Autodesk Fusion 360 part; units mm, degrees
note: some values were not read from the file. Set by a fixed rule: which sketch regions a step uses.
(part 4 of 7)
sketch "Sketch76" plane through (0, 116.2145, -31.1396) normal (0, 0.965926, -0.258819) x (-1, 0, 0)
  line L0 (-35.9419, 179.9959) -> (-35.9419, 150.9959)
  line L1 (-35.9419, 150.9959) -> (-72.9419, 150.9959)
  line L2 (-72.9419, 150.9959) -> (-72.9419, 179.9959)
  line L3 (-72.9419, 179.9959) -> (-35.9419, 179.9959)
  line L4 (-30, -37.2933) -> (-30, -46.5838)
  line L5 (-30, -46.5838) -> (22.741, -46.5838)
  ellipse E0 centre (22.741, -39.3535) end of major axis (22.741, -46.5838) minor radius 7 (22.741, -46.5838) -> (29.741, -39.3535) ccw
  line L6 (29.741, -39.3535) -> (29.741, 209.5755)
  ellipse E1 centre (22.741, 209.5755) end of major axis (22.741, 216.8058) minor radius 7 (29.741, 209.5755) -> (22.741, 216.8058) ccw
  line L7 (22.741, 216.8058) -> (-123.259, 216.8058)
  ellipse E2 centre (-123.259, 209.5755) end of major axis (-123.259, 216.8058) minor radius 7 (-123.259, 216.8058) -> (-130.259, 209.5755) ccw
  line L8 (-130.259, 209.5755) -> (-130.259, -39.3535)
  ellipse E3 centre (-123.259, -39.3535) end of major axis (-123.259, -46.5838) minor radius 7 (-130.259, -39.3535) -> (-123.259, -46.5838) ccw
  line L9 (-60.0369, -46.5838) -> (-60.0369, -37.2933)
  line L10 (-10, 70) -> (10, 70)
  arc A0 (20, 60) -> (10, 70) centre (10, 60) ccw
  line L11 (20, 60) -> (20, 40)
  arc A1 (10, 30) -> (20, 40) centre (10, 40) ccw
  line L12 (10, 30) -> (-10, 30)
  arc A2 (-20, 40) -> (-10, 30) centre (-10, 40) ccw
  line L13 (-20, 40) -> (-20, 60)
  arc A3 (-10, 70) -> (-20, 60) centre (-10, 60) ccw
  line L14 (-40, 30) -> (-110, 30)
  arc A4 (-120, 40) -> (-110, 30) centre (-110, 40) ccw
  line L15 (-120, 40) -> (-120, 60)
  arc A5 (-110, 70) -> (-120, 60) centre (-110, 60) ccw
  line L16 (-110, 70) -> (-40, 70)
  arc A6 (-30, 60) -> (-40, 70) centre (-40, 60) ccw
  line L17 (-30, 60) -> (-30, 40)
  arc A7 (-40, 30) -> (-30, 40) centre (-40, 40) ccw
  line L18 (22.9316, 100) -> (22.9316, 85)
  arc A8 (12.9316, 75) -> (22.9316, 85) centre (12.9316, 85) ccw
  line L19 (12.9316, 75) -> (7.9281, 75)
  arc A9 (-2.0719, 85) -> (7.9281, 75) centre (7.9281, 85) ccw
  line L20 (-2.0719, 85) -> (-2.0719, 100)
  arc A10 (7.9281, 110) -> (-2.0719, 100) centre (7.9281, 100) ccw
  line L21 (7.9281, 110) -> (12.9316, 110)
  arc A11 (22.9316, 100) -> (12.9316, 110) centre (12.9316, 100) ccw
  line L22 (-45.44, 85) -> (-45.44, 100)
  arc A12 (-35.44, 110) -> (-45.44, 100) centre (-35.44, 100) ccw
  line L23 (-35.44, 110) -> (-20, 110)
  arc A13 (-10, 100) -> (-20, 110) centre (-20, 100) ccw
  line L24 (-10, 100) -> (-10, 85)
  arc A14 (-20, 75) -> (-10, 85) centre (-20, 85) ccw
  line L25 (-20, 75) -> (-35.44, 75)
  arc A15 (-45.44, 85) -> (-35.44, 75) centre (-35.44, 85) ccw
  line L26 (-120, 85) -> (-120, 100)
  arc A16 (-110, 110) -> (-120, 100) centre (-110, 100) ccw
  line L27 (-110, 110) -> (-61.6636, 110)
  arc A17 (-51.6636, 100) -> (-61.6636, 110) centre (-61.6636, 100) ccw
  line L28 (-51.6636, 100) -> (-51.6636, 85)
  arc A18 (-61.6636, 75) -> (-51.6636, 85) centre (-61.6636, 85) ccw
  line L29 (-61.6636, 75) -> (-110, 75)
  arc A19 (-120, 85) -> (-110, 75) centre (-110, 85) ccw
  arc A20 (-76.4093, 196.948) -> (-80.3534, 201.8353) centre (-81.4093, 196.948) ccw
  line L30 (-76.4093, 196.948) -> (-76.4093, 176.5782)
  line L31 (-76.4093, 176.5782) -> (-84.2974, 176.5782)
  line L32 (-84.2974, 176.5782) -> (-84.2974, 196.948)
  arc A21 (-80.3534, 201.8353) -> (-84.2974, 196.948) centre (-79.2974, 196.948) ccw
  arc A22 (-84.2974, 121.8844) -> (-80.3534, 116.9972) centre (-79.2974, 121.8844) ccw
  line L33 (-84.2974, 121.8844) -> (-84.2974, 171.0352)
  line L34 (-84.2974, 171.0352) -> (-76.4093, 171.0352)
  line L35 (-76.4093, 171.0352) -> (-76.4093, 121.8844)
  arc A23 (-80.3534, 116.9972) -> (-76.4093, 121.8844) centre (-81.4093, 121.8844) ccw
  line L36 (-37.5, 135) -> (-67.5, 135)
  arc A24 (-70, 137.5) -> (-67.5, 135) centre (-67.5, 137.5) ccw
  line L37 (-70, 137.5) -> (-70, 142.5)
  arc A25 (-67.5, 145) -> (-70, 142.5) centre (-67.5, 142.5) ccw
  line L38 (-67.5, 145) -> (-37.5, 145)
  arc A26 (-35, 142.5) -> (-37.5, 145) centre (-37.5, 142.5) ccw
  line L39 (-35, 142.5) -> (-35, 137.5)
  arc A27 (-37.5, 135) -> (-35, 137.5) centre (-37.5, 137.5) ccw
  arc A28 (-90.5983, 197.0502) -> (-95.5983, 202.0502) centre (-95.5983, 197.0502) ccw
  line L40 (-90.5983, 197.0502) -> (-90.5983, 159.5626)
  line L41 (-90.5983, 159.5626) -> (-100.6526, 159.5626)
  line L42 (-100.6526, 159.5626) -> (-100.6526, 197.0502)
  arc A29 (-95.6526, 202.0502) -> (-100.6526, 197.0502) centre (-95.6526, 197.0502) ccw
  line L43 (-95.6526, 202.0502) -> (-95.5983, 202.0502)
  line L44 (-95.5983, 117.0948) -> (-95.6526, 117.0948)
  arc A30 (-100.6526, 122.0948) -> (-95.6526, 117.0948) centre (-95.6526, 122.0948) ccw
  line L45 (-100.6526, 122.0948) -> (-100.6526, 154.3733)
  line L46 (-100.6526, 154.3733) -> (-90.5983, 154.3733)
  line L47 (-90.5983, 154.3733) -> (-90.5983, 122.0948)
  arc A31 (-95.5983, 117.0948) -> (-90.5983, 122.0948) centre (-95.5983, 122.0948) ccw
  line L48 (-35, 125) -> (-35, 117.5)
  arc A32 (-37.5, 115) -> (-35, 117.5) centre (-37.5, 117.5) ccw
  line L49 (-37.5, 115) -> (-65, 115)
  arc A33 (-70, 120) -> (-65, 115) centre (-65, 120) ccw
  line L50 (-70, 120) -> (-70, 125)
  arc A34 (-65, 130) -> (-70, 125) centre (-65, 125) ccw
  line L51 (-65, 130) -> (-40, 130)
  arc A35 (-35, 125) -> (-40, 130) centre (-40, 125) ccw
  line L52 (-109.8689, 117.075) -> (-111.5449, 117.075)
  arc A36 (-116.5449, 122.075) -> (-111.5449, 117.075) centre (-111.5449, 122.075) ccw
  line L53 (-116.5449, 122.075) -> (-116.5449, 197.0502)
  arc A37 (-111.5449, 202.0502) -> (-116.5449, 197.0502) centre (-111.5449, 197.0502) ccw
  line L54 (-111.5449, 202.0502) -> (-109.8689, 202.0502)
  arc A38 (-104.8689, 197.0502) -> (-109.8689, 202.0502) centre (-109.8689, 197.0502) ccw
  line L55 (-104.8689, 197.0502) -> (-104.8689, 122.075)
  arc A39 (-109.8689, 117.075) -> (-104.8689, 122.075) centre (-109.8689, 122.075) ccw
  line L56 (25, 165) -> (0, 155)
  line L57 (0, 155) -> (0, 160)
  line L58 (0, 160) -> (25, 170)
  line L59 (25, 170) -> (25, 165)
  line L60 (25, 205) -> (0, 195)
  line L61 (0, 195) -> (0, 200)
  line L62 (0, 200) -> (25, 210)
  line L63 (25, 210) -> (25, 205)
  line L64 (-30, 170) -> (-30, 175)
  line L65 (-30, 175) -> (-5, 170)
  line L66 (-5, 170) -> (-5, 165)
  line L67 (-5, 165) -> (-30, 170)
  line L68 (-30, 180) -> (-30, 184.9041)
  line L69 (-30, 184.9041) -> (-5, 180)
  line L70 (-5, 180) -> (-5, 175)
  line L71 (-5, 175) -> (-30, 180)
  line L72 (25, 195) -> (0, 185)
  line L73 (0, 185) -> (0, 190)
  line L74 (0, 190) -> (25, 200)
  line L75 (25, 200) -> (25, 195)
  line L76 (25, 155) -> (0, 145)
  line L77 (0, 145) -> (0, 150)
  line L78 (0, 150) -> (25, 160)
  line L79 (25, 160) -> (25, 155)
  line L80 (25, 180.1705) -> (25, 175)
  line L81 (25, 175) -> (0, 165)
  line L82 (0, 165) -> (0, 170)
  line L83 (0, 170) -> (25, 180.1705)
  line L84 (-30, 200) -> (-30, 205)
  line L85 (-30, 205) -> (-5, 200)
  line L86 (-5, 200) -> (-5, 195)
  line L87 (-5, 195) -> (-30, 200)
  line L88 (-30, 160) -> (-30, 165.149)
  line L89 (-30, 165.149) -> (-5, 160.149)
  line L90 (-5, 160.149) -> (-5, 155)
  line L91 (-5, 155) -> (-30, 160)
  line L92 (-30, 150) -> (-30, 155)
  line L93 (-30, 155) -> (-5, 150)
  line L94 (-5, 150) -> (-5, 145)
  line L95 (-5, 145) -> (-30, 150)
  line L96 (-5, 190) -> (-5, 184.9041)
  line L97 (-5, 184.9041) -> (-30, 189.9041)
  line L98 (-30, 189.9041) -> (-30, 195)
  line L99 (-30, 195) -> (-5, 190)
  line L100 (25, 185) -> (0, 175)
  line L101 (0, 175) -> (0, 180.1897)
  line L102 (0, 180.1897) -> (25, 190.1897)
  line L103 (25, 190.1897) -> (25, 185)
  line L104 (-55, 204.5671) -> (-55, 201.6)
  arc A40 (-56.6, 200) -> (-55, 201.6) centre (-56.6, 201.6) ccw
  line L105 (-56.6, 200) -> (-68.7895, 200)
  arc A41 (-70.3895, 201.6) -> (-68.7895, 200) centre (-68.7895, 201.6) ccw
  line L106 (-70.3895, 201.6) -> (-70.3895, 204.5671)
  arc A42 (-68.7895, 206.1671) -> (-70.3895, 204.5671) centre (-68.7895, 204.5671) ccw
  line L107 (-68.7895, 206.1671) -> (-56.6, 206.1671)
  arc A43 (-55, 204.5671) -> (-56.6, 206.1671) centre (-56.6, 204.5671) ccw
  line L108 (-35, 204.6984) -> (-35, 201.6)
  arc A44 (-36.6, 200) -> (-35, 201.6) centre (-36.6, 201.6) ccw
  line L109 (-36.6, 200) -> (-48.311, 200)
  arc A45 (-49.911, 201.6) -> (-48.311, 200) centre (-48.311, 201.6) ccw
  line L110 (-49.911, 201.6) -> (-49.911, 204.6984)
  arc A46 (-48.311, 206.2984) -> (-49.911, 204.6984) centre (-48.311, 204.6984) ccw
  line L111 (-48.311, 206.2984) -> (-36.6, 206.2984)
  arc A47 (-35, 204.6984) -> (-36.6, 206.2984) centre (-36.6, 204.6984) ccw
  line L112 (-55, 195.348) -> (-55, 186.6)
  arc A48 (-56.6, 185) -> (-55, 186.6) centre (-56.6, 186.6) ccw
  line L113 (-56.6, 185) -> (-68.3957, 185)
  arc A49 (-69.9957, 186.6) -> (-68.3957, 185) centre (-68.3957, 186.6) ccw
  line L114 (-69.9957, 186.6) -> (-69.9957, 195.348)
  arc A50 (-68.3957, 196.948) -> (-69.9957, 195.348) centre (-68.3957, 195.348) ccw
  line L115 (-68.3957, 196.948) -> (-56.6, 196.948)
  arc A51 (-55, 195.348) -> (-56.6, 196.948) centre (-56.6, 195.348) ccw
  line L116 (-36.6, 185) -> (-48.311, 185)
  arc A52 (-49.911, 186.6) -> (-48.311, 185) centre (-48.311, 186.6) ccw
  line L117 (-49.911, 186.6) -> (-49.911, 195.348)
  arc A53 (-48.311, 196.948) -> (-49.911, 195.348) centre (-48.311, 195.348) ccw
  line L118 (-48.311, 196.948) -> (-36.6, 196.948)
  arc A54 (-35, 195.348) -> (-36.6, 196.948) centre (-36.6, 195.348) ccw
  line L119 (-35, 195.348) -> (-35, 186.6)
  arc A55 (-36.6, 185) -> (-35, 186.6) centre (-36.6, 186.6) ccw
  line L120 (-36.1991, 10) -> (-55, 10)
  line L121 (-55, 10) -> (-55, 30)
  line L122 (-55, 30) -> (-36.1991, 30)
  line L123 (-36.1991, 30) -> (-36.1991, 10)
  line L124 (-36.1991, -37.2933) -> (-30, -37.2933)
  line L125 (-123.259, -46.5838) -> (-60.0369, -46.5838)
  line L126 (-60, -37.2933) -> (-60, 10)
  line L127 (-60, 10) -> (-36.1991, 10)
  line L128 (-36.1991, 10) -> (-36.1991, -37.2933)
  line L129 (-60.0369, -37.2933) -> (-60, -37.2933)
  constraint horizontal L120
  constraint vertical L121
  constraint horizontal L122
  constraint vertical L123
  constraint coincident L14 L121.end
sketch "Sketch77" plane through (36.1991, 0, 0) normal (1, 0, 0) x (0, 0, -1)
  line L0 (66.3857, 103.6645) -> (67.1622, 106.5623)
  line L1 (67.1622, 106.5623) -> (2.1618, 123.9791)
  line L2 (2.1618, 123.9791) -> (1.3854, 121.0813)
  line L3 (1.3854, 121.0813) -> (66.3857, 103.6645)
  line L4 (2.1618, 123.9791) -> (4.8748, 123.2521)
  line L5 (4.0841, 120.3582) -> (4.8748, 123.2521)
  line L6 (4.0841, 120.3582) -> (1.3854, 121.0813)
  line L7 (1.3854, 121.0813) -> (2.1618, 123.9791)
  constraint coincident L1.end L2.start
  constraint coincident L1 L4.end
  constraint coincident L3 L5.start
  constraint coincident L2.end L3.start
sketch "Sketch78" plane through (30, 0, 0) normal (1, 0, 0) x (0, 0, -1)
  line L0 (66.3857, 103.6645) -> (73.1159, 101.8612)
  line L1 (73.1159, 101.8612) -> (73.1008, 100.1316)
  line L2 (73.1008, 100.1316) -> (76.1007, 100.1054)
  line L3 (76.1007, 100.1054) -> (76.136, 104.1577)
  line L4 (76.136, 104.1577) -> (67.1622, 106.5623)
  line L5 (67.1622, 106.5623) -> (66.3857, 103.6645)
sketch "Sketch79" plane through (30, 0, 0) normal (1, 0, 0) x (0, 0, -1)
  line L0 (66.8047, 105.612) -> (72.4158, 104.2598)
  line L1 (72.4158, 104.2598) -> (71.9146, 102.1798)
  line L2 (71.9146, 102.1798) -> (66.194, 103.7808)
  line L3 (66.194, 103.7808) -> (66.8047, 105.612)
  constraint perpendicular L0 L1
sketch "Sketch80" plane through (60.0369, 0, 0) normal (-1, 0, 0) x (0, 0, 1)
  line L0 (-67.1622, 106.5623) -> (-76.136, 104.1577)
  line L1 (-76.136, 104.1577) -> (-76.1007, 100.1054)
  line L2 (-76.1007, 100.1054) -> (-73.1008, 100.1316)
  line L3 (-73.1008, 100.1316) -> (-73.1159, 101.8612)
  line L4 (-73.1159, 101.8612) -> (-66.3857, 103.6645)
  line L5 (-66.3857, 103.6645) -> (-67.1622, 106.5623)
  line L6 (-67.1622, 106.5623) -> (-73.5344, 104.8549)
  line L7 (-73.5344, 104.8549) -> (-73.1159, 101.8612)
  line L8 (-66.3857, 103.6645) -> (-67.1622, 106.5623)
  line L9 (-66.3857, 103.6645) -> (-73.1159, 101.8612)
  constraint coincident L0.start L5.end
  constraint perpendicular L5 L6
  constraint coincident L3.end L4.start
  constraint coincident L4.end L5.start
move_body "Move10" bodies 1 to x (1, 0, 0) y (0, 0.996195, 0.087156) z (0, -0.087156, 0.996195) at (0, -2.7665, -9.3244) in component "axe"
move_body "Move11" bodies 1 to x (1, 0, 0) y (0, 0.939693, 0.34202) z (0, -0.34202, 0.939693) at (0, -8.7094, -41.4265) in component "axe"
move_body "Move12" bodies 1 to x (1, 0, 0) y (0, 0.866025, -0.5) z (0, 0.5, 0.866025) at (0, 33.3731, 55.0959) in component "axe"
sketch "Sketch82" plane through (0, 114.2827, -30.6219) normal (0, 0.965926, -0.258819) x (-1, 0, 0)
  arc A0 (-118, 34) -> (-111.9229, 30.1866) centre (-110, 40) ccw
  line L0 (-111.9229, 30.1866) -> (-65, 70)
  line L1 (-65, 70) -> (-75.5714, 70)
  line L2 (-75.5714, 70) -> (-118, 34)
  line L3 (-30, 70) -> (-124.0059, 70)
  line L4 (-124.0059, 70) -> (-124.0059, 27.6298)
  line L5 (-124.0059, 27.6298) -> (-30, 27.6298)
  line L6 (-30, 27.6298) -> (-30, 70)
  line L7 (-50, 70) -> (22.4251, 70)
  line L8 (22.4251, 70) -> (22.4251, 27.6298)
  line L9 (22.4251, 27.6298) -> (-50, 27.6298)
  line L10 (-50, 27.6298) -> (-50, 70)
  constraint horizontal L3
  constraint vertical L4
  constraint horizontal L5
  constraint vertical L6
  constraint horizontal L7
  constraint vertical L8
  constraint horizontal L9
  constraint vertical L10
  constraint coincident L3 L7.start
sketch "Sketch83" plane through (0, 114.2827, -30.6219) normal (0, 0.965926, -0.258819) x (-1, 0, 0)
  line L0 (-50, 51.191) -> (-50, 40.2326)
  line L1 (-50, 40.2326) -> (-30, 58.8372)
  line L2 (-30, 58.8372) -> (-30, 60)
  arc A0 (-30, 60) -> (-32.9289, 67.0711) centre (-40, 60) ccw
  line L3 (-32.9289, 67.0711) -> (-50, 51.191)
  line L4 (-52.9181, 73.2158) -> (-27.1295, 73.2158)
  line L5 (-27.1295, 73.2158) -> (-27.1295, 28.4672)
  line L6 (-27.1295, 28.4672) -> (-52.9181, 28.4672)
  line L7 (-52.9181, 28.4672) -> (-52.9181, 73.2158)
  constraint horizontal L4
  constraint vertical L5
  constraint horizontal L6
  constraint vertical L7
sketch "Sketch84" plane through (0, 114.7656, -30.7514) normal (0, 0.965926, -0.258819) x (-1, 0, 0)
  arc A0 (-18, 66) -> (-20, 60) centre (-10, 60) ccw
  line L0 (-20, 60) -> (-20, 50)
  line L1 (-20, 50) -> (-2, 52)
  line L2 (-2, 52) -> (-18, 66)
  line L3 (-49.6341, 112.7411) -> (24.709, 112.7411)
  line L4 (24.709, 112.7411) -> (24.709, 27.7535)
  line L5 (24.709, 27.7535) -> (-49.6341, 27.7535)
  line L6 (-49.6341, 27.7535) -> (-49.6341, 112.7411)
  constraint horizontal L3
  constraint vertical L4
  constraint horizontal L5
  constraint vertical L6
sketch "Sketch85" plane through (0, 115.0071, -30.8161) normal (0, 0.965926, -0.258819) x (-1, 0, 0)
  line L0 (-124.1638, 112.0554) -> (-45, 112.0554)
  line L1 (-45, 112.0554) -> (-45, 70)
  line L2 (-45, 70) -> (-124.1638, 70)
  line L3 (-124.1638, 70) -> (-124.1638, 112.0554)
  line L4 (-75, 115) -> (-120, 115)
  line L5 (-120, 115) -> (-120, 205)
  line L6 (-120, 205) -> (-75, 205)
  line L7 (-75, 205) -> (-75, 115)
  line L8 (-31.9508, 112.0554) -> (-75, 112.0554)
  line L9 (-75, 112.0554) -> (-75, 147.4067)
  line L10 (-75, 147.4067) -> (-31.9508, 147.4067)
  line L11 (-31.9508, 147.4067) -> (-31.9508, 112.0554)
  constraint horizontal L0
  constraint vertical L1
  constraint horizontal L2
  constraint vertical L3
  constraint horizontal L4
  constraint vertical L5
  constraint horizontal L6
  constraint vertical L7
  constraint horizontal L8
  constraint vertical L9
  constraint horizontal L10
  constraint vertical L11
  constraint coincident L7 L9.end
sketch "Sketch86" plane through (0, 115.2486, -30.8808) normal (0, 0.965926, -0.258819) x (-1, 0, 0)
  arc A0 (-56.6, 185) -> (-55, 186.6) centre (-56.6, 186.6) ccw
  line L0 (-55, 186.6) -> (-55, 195.348)
  arc A1 (-55, 195.348) -> (-56.6, 196.948) centre (-56.6, 195.348) ccw
  line L1 (-56.6, 196.948) -> (-68.3957, 196.948)
  arc A2 (-68.3957, 196.948) -> (-69.9957, 195.348) centre (-68.3957, 195.348) ccw
  line L2 (-69.9957, 195.348) -> (-69.9957, 186.6)
  arc A3 (-69.9957, 186.6) -> (-68.3957, 185) centre (-68.3957, 186.6) ccw
  line L3 (-68.3957, 185) -> (-56.6, 185)
  line L4 (-73.6191, 208.4794) -> (-32.1874, 208.4794)
  line L5 (-32.1874, 208.4794) -> (-32.1874, 182.1137)
  line L6 (-32.1874, 182.1137) -> (-73.6191, 182.1137)
  line L7 (-73.6191, 182.1137) -> (-73.6191, 208.4794)
  constraint horizontal L4
  constraint vertical L5
  constraint horizontal L6
  constraint vertical L7
sketch "Sketch87" plane through (0, 116.2145, -31.1396) normal (0, 0.965926, -0.258819) x (-1, 0, 0)
  line L0 (-55, 27.1913) -> (-36.1991, 27.1913)
  line L1 (-36.1991, 27.1913) -> (-36.1991, -37.2933)
  line L2 (-30, -37.2933) -> (-30, -46.5838)
  line L3 (-30, -46.5838) -> (22.741, -46.5838)
  ellipse E0 centre (22.741, -39.3535) end of major axis (22.741, -46.5838) minor radius 7 (22.741, -46.5838) -> (29.741, -39.3535) ccw
  line L4 (29.741, -39.3535) -> (29.741, 209.5755)
  ellipse E1 centre (22.741, 209.5755) end of major axis (22.741, 216.8058) minor radius 7 (29.741, 209.5755) -> (22.741, 216.8058) ccw
  line L5 (22.741, 216.8058) -> (-123.259, 216.8058)
  ellipse E2 centre (-123.259, 209.5755) end of major axis (-123.259, 216.8058) minor radius 7 (-123.259, 216.8058) -> (-130.259, 209.5755) ccw
  line L6 (-130.259, 209.5755) -> (-130.259, -39.3535)
  ellipse E3 centre (-123.259, -39.3535) end of major axis (-123.259, -46.5838) minor radius 7 (-130.259, -39.3535) -> (-123.259, -46.5838) ccw
  line L7 (-123.259, -46.5838) -> (-60.0369, -46.5838)
  line L8 (-60.0369, -46.5838) -> (-60.0369, -43.8903)
  line L9 (-55, 10) -> (-55, 27.1913)
  line L10 (25, 180.1705) -> (25, 175)
  line L11 (25, 175) -> (0, 165)
  line L12 (0, 165) -> (0, 170)
  line L13 (0, 170) -> (25, 180.1705)
  line L14 (-30, 200) -> (-30, 205)
  line L15 (-30, 205) -> (-5, 200)
  line L16 (-5, 200) -> (-5, 195)
  line L17 (-5, 195) -> (-30, 200)
  line L18 (-30, 160) -> (-30, 165.149)
  line L19 (-30, 165.149) -> (-5, 160.149)
  line L20 (-5, 160.149) -> (-5, 155)
  line L21 (-5, 155) -> (-30, 160)
  line L22 (-30, 170) -> (-30, 175)
  line L23 (-30, 175) -> (-5, 170)
  line L24 (-5, 170) -> (-5, 165)
  line L25 (-5, 165) -> (-30, 170)
  line L26 (25, 205) -> (0, 195)
  line L27 (0, 195) -> (0, 200)
  line L28 (0, 200) -> (25, 210)
  line L29 (25, 210) -> (25, 205)
  line L30 (25, 165) -> (0, 155)
  line L31 (0, 155) -> (0, 160)
  line L32 (0, 160) -> (25, 170)
  line L33 (25, 170) -> (25, 165)
  line L34 (25, 185) -> (0, 175)
  line L35 (0, 175) -> (0, 180.1897)
  line L36 (0, 180.1897) -> (25, 190.1897)
  line L37 (25, 190.1897) -> (25, 185)
  line L38 (-5, 190) -> (-5, 184.9041)
  line L39 (-5, 184.9041) -> (-30, 189.9041)
  line L40 (-30, 189.9041) -> (-30, 195)
  line L41 (-30, 195) -> (-5, 190)
  line L42 (-30, 150) -> (-30, 155)
  line L43 (-30, 155) -> (-5, 150)
  line L44 (-5, 150) -> (-5, 145)
  line L45 (-5, 145) -> (-30, 150)
  line L46 (-30, 180) -> (-30, 184.9041)
  line L47 (-30, 184.9041) -> (-5, 180)
  line L48 (-5, 180) -> (-5, 175)
  line L49 (-5, 175) -> (-30, 180)
  line L50 (25, 195) -> (0, 185)
  line L51 (0, 185) -> (0, 190)
  line L52 (0, 190) -> (25, 200)
  line L53 (25, 200) -> (25, 195)
  line L54 (25, 155) -> (0, 145)
  line L55 (0, 145) -> (0, 150)
  line L56 (0, 150) -> (25, 160)
  line L57 (25, 160) -> (25, 155)
  line L58 (-35.9419, 179.9959) -> (-35.9419, 150.9959)
  line L59 (-35.9419, 150.9959) -> (-72.9419, 150.9959)
  line L60 (-72.9419, 150.9959) -> (-72.9419, 179.9959)
  line L61 (-72.9419, 179.9959) -> (-35.9419, 179.9959)
  line L62 (-68.2863, 161.1701) -> (-19.9788, 161.1701) construction
  line L63 (-19.9788, 161.1701) -> (-19.9788, 204.0599) construction
  line L64 (-19.9788, 204.0599) -> (-68.2863, 204.0599) construction
  line L65 (-68.2863, 204.0599) -> (-68.2863, 161.1701) construction
  line L66 (-36.1991, -37.2933) -> (-30, -37.2933)
  line L67 (-60.0369, -43.8903) -> (-55.0369, -43.8903)
  line L68 (-55.0369, -43.8903) -> (-55.0369, -37.2933)
  line L69 (-55.0369, -37.2933) -> (-60, -37.2933)
  line L70 (-60, -37.2933) -> (-60, 10)
  line L71 (-60, 10) -> (-55, 10)
  dimension "d317" = 6.5
sketch "Sketch88" plane through (0, 116.2145, -31.1396) normal (0, 0.965926, -0.258819) x (-1, 0, 0)
  line L0 (-35.9419, 179.9959) -> (-35.9419, 150.9959)
  line L1 (-35.9419, 150.9959) -> (-72.9419, 150.9959)
  line L2 (-72.9419, 150.9959) -> (-72.9419, 179.9959)
  line L3 (-72.9419, 179.9959) -> (-35.9419, 179.9959)
  line L4 (25, 155) -> (0, 145)
  line L5 (0, 145) -> (0, 150)
  line L6 (0, 150) -> (25, 160)
  line L7 (25, 160) -> (25, 155)
  line L8 (25, 195) -> (0, 185)
  line L9 (0, 185) -> (0, 190)
  line L10 (0, 190) -> (25, 200)
  line L11 (25, 200) -> (25, 195)
  line L12 (-30, 180) -> (-30, 184.9041)
  line L13 (-30, 184.9041) -> (-5, 180)
  line L14 (-5, 180) -> (-5, 175)
  line L15 (-5, 175) -> (-30, 180)
  line L16 (-30, 150) -> (-30, 155)
  line L17 (-30, 155) -> (-5, 150)
  line L18 (-5, 150) -> (-5, 145)
  line L19 (-5, 145) -> (-30, 150)
  line L20 (-5, 190) -> (-5, 184.9041)
  line L21 (-5, 184.9041) -> (-30, 189.9041)
  line L22 (-30, 189.9041) -> (-30, 195)
  line L23 (-30, 195) -> (-5, 190)
  line L24 (25, 185) -> (0, 175)
  line L25 (0, 175) -> (0, 180.1897)
  line L26 (0, 180.1897) -> (25, 190.1897)
  line L27 (25, 190.1897) -> (25, 185)
  line L28 (25, 165) -> (0, 155)
  line L29 (0, 155) -> (0, 160)
  line L30 (0, 160) -> (25, 170)
  line L31 (25, 170) -> (25, 165)
  line L32 (25, 205) -> (0, 195)
  line L33 (0, 195) -> (0, 200)
  line L34 (0, 200) -> (25, 210)
  line L35 (25, 210) -> (25, 205)
  line L36 (-30, 170) -> (-30, 175)
  line L37 (-30, 175) -> (-5, 170)
  line L38 (-5, 170) -> (-5, 165)
  line L39 (-5, 165) -> (-30, 170)
  line L40 (-30, 160) -> (-30, 165.149)
  line L41 (-30, 165.149) -> (-5, 160.149)
  line L42 (-5, 160.149) -> (-5, 155)
  line L43 (-5, 155) -> (-30, 160)
  line L44 (-30, 200) -> (-30, 205)
  line L45 (-30, 205) -> (-5, 200)
  line L46 (-5, 200) -> (-5, 195)
  line L47 (-5, 195) -> (-30, 200)
  line L48 (25, 180.1705) -> (25, 175)
  line L49 (25, 175) -> (0, 165)
  line L50 (0, 165) -> (0, 170)
  line L51 (0, 170) -> (25, 180.1705)
  line L52 (-55, 27.1913) -> (-36.1991, 27.1913)
  line L53 (-36.1991, 27.1913) -> (-36.1991, -37.2933)
  line L54 (-30, -37.2933) -> (-30, -46.5838)
  line L55 (-30, -46.5838) -> (22.741, -46.5838)
  ellipse E0 centre (22.741, -39.3535) end of major axis (22.741, -46.5838) minor radius 7 (22.741, -46.5838) -> (29.741, -39.3535) ccw
  line L56 (29.741, -39.3535) -> (29.741, 209.5755)
  ellipse E1 centre (22.741, 209.5755) end of major axis (22.741, 216.8058) minor radius 7 (29.741, 209.5755) -> (22.741, 216.8058) ccw
  line L57 (22.741, 216.8058) -> (-123.259, 216.8058)
  ellipse E2 centre (-123.259, 209.5755) end of major axis (-123.259, 216.8058) minor radius 7 (-123.259, 216.8058) -> (-130.259, 209.5755) ccw
  line L58 (-130.259, 209.5755) -> (-130.259, -39.3535)
  ellipse E3 centre (-123.259, -39.3535) end of major axis (-123.259, -46.5838) minor radius 7 (-130.259, -39.3535) -> (-123.259, -46.5838) ccw
  line L59 (-123.259, -46.5838) -> (-60.0369, -46.5838)
  line L60 (-60.0369, -46.5838) -> (-60.0369, -43.8903)
  line L61 (-55, 10) -> (-55, 27.1913)
  line L62 (-63.1164, 198.8989) -> (-63.1164, 200.1093)
  line L63 (-63.1164, 200.1093) -> (-65.0274, 200.1093)
  line L64 (-65.0274, 200.1093) -> (-65.0274, 200.872)
  line L65 (-65.0274, 200.872) -> (-62.274, 200.8764)
  line L66 (-62.274, 200.8764) -> (-62.274, 198.4644)
  spline S0 degree 3 poles (-62.274, 198.4644) (-62.4834, 198.3077) (-62.8901, 198.0035) (-63.356, 197.8018) (-63.582, 197.704) knots 0 0 0 0 0.078157 0.151758 0.151758 0.151758 0.151758
  spline S1 degree 3 poles (-63.582, 197.704) (-63.8076, 197.6296) (-64.2571, 197.4815) (-64.7299, 197.4598) (-64.9653, 197.449) knots 0 0 0 0 0.070908 0.141252 0.141252 0.141252 0.141252
  spline S2 degree 3 poles (-64.9653, 197.449) (-65.2744, 197.4647) (-65.8798, 197.4952) (-66.4342, 197.7396) (-66.7056, 197.8592) knots 0 0 0 0 0.091966 0.180141 0.180141 0.180141 0.180141
  spline S3 degree 3 poles (-66.7056, 197.8592) (-66.9503, 198.0107) (-67.4379, 198.3127) (-67.7378, 198.8016) (-67.8872, 199.0452) knots 0 0 0 0 0.085037 0.169503 0.169503 0.169503 0.169503
  spline S4 degree 3 poles (-67.8872, 199.0452) (-68.0036, 199.3151) (-68.2421, 199.8684) (-68.2713, 200.4705) (-68.2863, 200.7789) knots 0 0 0 0 0.087419 0.179189 0.179189 0.179189 0.179189
  spline S5 degree 3 poles (-68.2863, 200.7789) (-68.2704, 201.0885) (-68.239, 201.7016) (-68.0052, 202.2692) (-67.8895, 202.5502) knots 0 0 0 0 0.09226 0.182704 0.182704 0.182704 0.182704
  spline S6 degree 3 poles (-67.8895, 202.5502) (-67.7454, 202.8052) (-67.4631, 203.3049) (-66.9829, 203.6183) (-66.7477, 203.7717) knots 0 0 0 0 0.086466 0.169395 0.169395 0.169395 0.169395
  spline S7 degree 3 poles (-66.7477, 203.7717) (-66.4845, 203.888) (-65.9383, 204.1295) (-65.3412, 204.1567) (-65.0319, 204.1707) knots 0 0 0 0 0.085548 0.177538 0.177538 0.177538 0.177538
  spline S8 degree 3 poles (-65.0319, 204.1707) (-64.8061, 204.1627) (-64.3702, 204.147) (-63.9566, 204.009) (-63.7571, 203.9424) knots 0 0 0 0 0.067359 0.130098 0.130098 0.130098 0.130098
  spline S9 degree 3 poles (-63.7571, 203.9424) (-63.58, 203.862) (-63.2405, 203.7078) (-62.9856, 203.4361) (-62.8637, 203.3061) knots 0 0 0 0 0.057702 0.110632 0.110632 0.110632 0.110632
  spline S10 degree 3 poles (-62.8637, 203.3061) (-62.7607, 203.1533) (-62.5397, 202.8254) (-62.4301, 202.445) (-62.3716, 202.242) knots 0 0 0 0 0.054958 0.117884 0.117884 0.117884 0.117884
  line L67 (-62.3716, 202.242) -> (-63.1475, 202.0292)
  spline S11 degree 3 poles (-63.1475, 202.0292) (-63.1952, 202.1803) (-63.2823, 202.4566) (-63.4397, 202.6995) (-63.5111, 202.8096) knots 0 0 0 0 0.047276 0.086437 0.086437 0.086437 0.086437
  spline S12 degree 3 poles (-63.5111, 202.8096) (-63.5945, 202.9008) (-63.7708, 203.0935) (-64.0072, 203.2052) (-64.1318, 203.264) knots 0 0 0 0 0.036726 0.077589 0.077589 0.077589 0.077589
  spline S13 degree 3 poles (-64.1318, 203.264) (-64.2723, 203.3138) (-64.562, 203.4164) (-64.8692, 203.4285) (-65.0274, 203.4347) knots 0 0 0 0 0.044449 0.091641 0.091641 0.091641 0.091641
  spline S14 degree 3 poles (-65.0274, 203.4347) (-65.2124, 203.4292) (-65.5614, 203.4188) (-65.8919, 203.3075) (-66.0472, 203.2552) knots 0 0 0 0 0.055163 0.104053 0.104053 0.104053 0.104053
  spline S15 degree 3 poles (-66.0472, 203.2552) (-66.1815, 203.1929) (-66.439, 203.0735) (-66.6434, 202.877) (-66.7411, 202.7829) knots 0 0 0 0 0.044061 0.084453 0.084453 0.084453 0.084453
  spline S16 degree 3 poles (-66.7411, 202.7829) (-66.8239, 202.6836) (-66.988, 202.4867) (-67.0971, 202.2549) (-67.1512, 202.14) knots 0 0 0 0 0.038631 0.076535 0.076535 0.076535 0.076535
  spline S17 degree 3 poles (-67.1512, 202.14) (-67.2236, 201.9325) (-67.3714, 201.509) (-67.39, 201.0607) (-67.3995, 200.8321) knots 0 0 0 0 0.06555 0.133782 0.133782 0.133782 0.133782
  spline S18 degree 3 poles (-67.3995, 200.8321) (-67.3911, 200.5625) (-67.3753, 200.0597) (-67.1874, 199.5938) (-67.1002, 199.3778) knots 0 0 0 0 0.080159 0.149513 0.149513 0.149513 0.149513
  spline S19 degree 3 poles (-67.1002, 199.3778) (-66.9899, 199.1956) (-66.7709, 198.8342) (-66.4087, 198.6166) (-66.229, 198.5087) knots 0 0 0 0 0.06285 0.12472 0.12472 0.12472 0.12472
  spline S20 degree 3 poles (-66.229, 198.5087) (-66.0352, 198.426) (-65.6469, 198.2601) (-65.2253, 198.2367) (-65.0141, 198.225) knots 0 0 0 0 0.062693 0.125611 0.125611 0.125611 0.125611
  spline S21 degree 3 poles (-65.0141, 198.225) (-64.8284, 198.2342) (-64.4544, 198.2527) (-64.1012, 198.3773) (-63.9234, 198.44) knots 0 0 0 0 0.055462 0.111696 0.111696 0.111696 0.111696
  spline S22 degree 3 poles (-63.9234, 198.44) (-63.7635, 198.5072) (-63.4759, 198.6281) (-63.227, 198.8156) (-63.1164, 198.8989) knots 0 0 0 0 0.051788 0.093147 0.093147 0.093147 0.093147
  spline S23 degree 3 poles (-54.9382, 198.3003) (-54.9002, 198.2836) (-54.8136, 198.2455) (-54.7187, 198.2437) (-54.6656, 198.2427) knots 0 0 0 0 0.012364 0.028114 0.028114 0.028114 0.028114
  spline S24 degree 3 poles (-54.6656, 198.2427) (-54.6141, 198.2445) (-54.4969, 198.2487) (-54.3806, 198.2647) (-54.3153, 198.2737) knots 0 0 0 0 0.015427 0.035185 0.035185 0.035185 0.035185
  line L68 (-54.3153, 198.2737) -> (-54.2, 197.5688)
  spline S25 degree 3 poles (-54.2, 197.5688) (-54.3061, 197.5481) (-54.5053, 197.5093) (-54.7082, 197.5015) (-54.803, 197.4978) knots 0 0 0 0 0.032364 0.060796 0.060796 0.060796 0.060796
  spline S26 degree 3 poles (-54.803, 197.4978) (-54.9335, 197.5003) (-55.1673, 197.5048) (-55.3821, 197.5953) (-55.4769, 197.6353) knots 0 0 0 0 0.038727 0.069335 0.069335 0.069335 0.069335
  spline S27 degree 3 poles (-55.4769, 197.6353) (-55.5503, 197.6834) (-55.6922, 197.7765) (-55.7742, 197.9249) (-55.8139, 197.9966) knots 0 0 0 0 0.025865 0.050076 0.050076 0.050076 0.050076
  spline S28 degree 3 poles (-55.8139, 197.9966) (-55.842, 198.112) (-55.917, 198.4208) (-55.9136, 198.7393) (-55.9115, 198.9388) knots 0 0 0 0 0.035512 0.095031 0.095031 0.095031 0.095031
  line L69 (-55.9115, 198.9388) -> (-55.9115, 201.6479)
  line L70 (-55.9115, 201.6479) -> (-56.4967, 201.6479)
  line L71 (-56.4967, 201.6479) -> (-56.4967, 202.2686)
  line L72 (-56.4967, 202.2686) -> (-55.9115, 202.2686)
  line L73 (-55.9115, 202.2686) -> (-55.9115, 203.4347)
  line L74 (-55.9115, 203.4347) -> (-55.1178, 203.9136)
  line L75 (-55.1178, 203.9136) -> (-55.1178, 202.2686)
  line L76 (-55.1178, 202.2686) -> (-54.3153, 202.2686)
  line L77 (-54.3153, 202.2686) -> (-54.3153, 201.6479)
  line L78 (-54.3153, 201.6479) -> (-55.1178, 201.6479)
  line L79 (-55.1178, 201.6479) -> (-55.1178, 198.8945)
  spline S29 degree 3 poles (-55.1178, 198.8945) (-55.119, 198.8004) (-55.1208, 198.6523) (-55.0878, 198.5082) (-55.0757, 198.4555) knots 0 0 0 0 0.028064 0.044226 0.044226 0.044226 0.044226
  spline S30 degree 3 poles (-55.0757, 198.4555) (-55.0592, 198.4246) (-55.0259, 198.3618) (-54.9677, 198.321) (-54.9382, 198.3003) knots 0 0 0 0 0.010363 0.020994 0.020994 0.020994 0.020994
  line L80 (-47.6823, 204.0599) -> (-47.6823, 203.1421)
  line L81 (-47.6823, 203.1421) -> (-48.4804, 203.1421)
  line L82 (-48.4804, 203.1421) -> (-48.4804, 204.0599)
  line L83 (-48.4804, 204.0599) -> (-47.6823, 204.0599)
  spline S31 degree 3 poles (-45.3434, 188.1557) (-45.3053, 188.139) (-45.2188, 188.1009) (-45.1239, 188.0991) (-45.0707, 188.0981) knots 0 0 0 0 0.012364 0.028115 0.028115 0.028115 0.028115
  spline S32 degree 3 poles (-45.0707, 188.0981) (-45.0193, 188.0999) (-44.902, 188.1041) (-44.7858, 188.1201) (-44.7205, 188.1291) knots 0 0 0 0 0.015427 0.035184 0.035184 0.035184 0.035184
  line L84 (-44.7205, 188.1291) -> (-44.6052, 187.4241)
  spline S33 degree 3 poles (-44.6052, 187.4241) (-44.7113, 187.4035) (-44.9105, 187.3647) (-45.1133, 187.3569) (-45.2082, 187.3532) knots 0 0 0 0 0.032364 0.060796 0.060796 0.060796 0.060796
  spline S34 degree 3 poles (-45.2082, 187.3532) (-45.3387, 187.3557) (-45.5725, 187.3602) (-45.7873, 187.4507) (-45.8821, 187.4907) knots 0 0 0 0 0.038727 0.069335 0.069335 0.069335 0.069335
  spline S35 degree 3 poles (-45.8821, 187.4907) (-45.9554, 187.5388) (-46.0974, 187.6319) (-46.1794, 187.7803) (-46.2191, 187.852) knots 0 0 0 0 0.025865 0.050076 0.050076 0.050076 0.050076
  spline S36 degree 3 poles (-46.2191, 187.852) (-46.2471, 187.9674) (-46.3222, 188.2761) (-46.3188, 188.5947) (-46.3166, 188.7942) knots 0 0 0 0 0.035512 0.095031 0.095031 0.095031 0.095031
  line L85 (-46.3166, 188.7942) -> (-46.3166, 191.5033)
  line L86 (-46.3166, 191.5033) -> (-46.9019, 191.5033)
  line L87 (-46.9019, 191.5033) -> (-46.9019, 192.124)
  line L88 (-46.9019, 192.124) -> (-46.3166, 192.124)
  line L89 (-46.3166, 192.124) -> (-46.3166, 193.2901)
  line L90 (-46.3166, 193.2901) -> (-45.523, 193.769)
  line L91 (-45.523, 193.769) -> (-45.523, 192.124)
  line L92 (-45.523, 192.124) -> (-44.7205, 192.124)
  line L93 (-44.7205, 192.124) -> (-44.7205, 191.5033)
  line L94 (-44.7205, 191.5033) -> (-45.523, 191.5033)
  line L95 (-45.523, 191.5033) -> (-45.523, 188.7499)
  spline S37 degree 3 poles (-45.523, 188.7499) (-45.5242, 188.6558) (-45.526, 188.5076) (-45.4929, 188.3636) (-45.4809, 188.3109) knots 0 0 0 0 0.028064 0.044226 0.044226 0.044226 0.044226
  spline S38 degree 3 poles (-45.4809, 188.3109) (-45.4644, 188.2799) (-45.4311, 188.2172) (-45.3729, 188.1764) (-45.3434, 188.1557) knots 0 0 0 0 0.010363 0.020994 0.020994 0.020994 0.020994
  line L96 (-67.1956, 190.3017) -> (-67.1956, 187.4153)
  line L97 (-67.1956, 187.4153) -> (-68.0557, 187.4153)
  line L98 (-68.0557, 187.4153) -> (-68.0557, 193.9153)
  line L99 (-68.0557, 193.9153) -> (-65.1737, 193.9153)
  spline S39 degree 3 poles (-65.1737, 193.9153) (-64.917, 193.9133) (-64.4685, 193.9099) (-64.0369, 193.791) (-63.8525, 193.7401) knots 0 0 0 0 0.076609 0.133783 0.133783 0.133783 0.133783
  spline S40 degree 3 poles (-63.8525, 193.7401) (-63.7085, 193.6693) (-63.4151, 193.5248) (-63.226, 193.2577) (-63.1297, 193.1216) knots 0 0 0 0 0.047344 0.096479 0.096479 0.096479 0.096479
  spline S41 degree 3 poles (-63.1297, 193.1216) (-63.0509, 192.9692) (-62.8917, 192.6617) (-62.8702, 192.3161) (-62.8593, 192.1417) knots 0 0 0 0 0.050884 0.102649 0.102649 0.102649 0.102649
  spline S42 degree 3 poles (-62.8593, 192.1417) (-62.8767, 191.9216) (-62.911, 191.4883) (-63.1765, 191.1447) (-63.3071, 190.9756) knots 0 0 0 0 0.064712 0.127351 0.127351 0.127351 0.127351
  spline S43 degree 3 poles (-63.3071, 190.9756) (-63.4898, 190.8304) (-63.8954, 190.5079) (-64.4084, 190.4206) (-64.6905, 190.3726) knots 0 0 0 0 0.068929 0.153084 0.153084 0.153084 0.153084
  spline S44 degree 3 poles (-64.6905, 190.3726) (-64.588, 190.322) (-64.4042, 190.2312) (-64.243, 190.1049) (-64.1717, 190.049) knots 0 0 0 0 0.034174 0.061288 0.061288 0.061288 0.061288
  spline S45 degree 3 poles (-64.1717, 190.049) (-64.0453, 189.9227) (-63.7798, 189.6574) (-63.5685, 189.347) (-63.4578, 189.1844) knots 0 0 0 0 0.053478 0.112342 0.112342 0.112342 0.112342
  line L100 (-63.4578, 189.1844) -> (-62.3272, 187.4153)
  line L101 (-62.3272, 187.4153) -> (-63.4091, 187.4153)
  line L102 (-63.4091, 187.4153) -> (-64.2692, 188.7676)
  spline S46 degree 3 poles (-64.2692, 188.7676) (-64.3816, 188.9413) (-64.5791, 189.2464) (-64.7964, 189.5377) (-64.89, 189.6632) knots 0 0 0 0 0.06204 0.108997 0.108997 0.108997 0.108997
  spline S47 degree 3 poles (-64.89, 189.6632) (-64.9633, 189.7549) (-65.0926, 189.9165) (-65.256, 190.043) (-65.3267, 190.0977) knots 0 0 0 0 0.035073 0.061797 0.061797 0.061797 0.061797
  spline S48 degree 3 poles (-65.3267, 190.0977) (-65.3903, 190.1357) (-65.514, 190.2097) (-65.652, 190.2507) (-65.7191, 190.2707) knots 0 0 0 0 0.022121 0.04303 0.04303 0.04303 0.04303
  spline S49 degree 3 poles (-65.7191, 190.2707) (-65.7833, 190.2796) (-65.942, 190.3018) (-66.1024, 190.3018) (-66.198, 190.3017) knots 0 0 0 0 0.019427 0.048036 0.048036 0.048036 0.048036
  line L103 (-66.198, 190.3017) -> (-67.1956, 190.3017)
  spline S50 degree 3 poles (-54.5192, 187.3089) (-54.7824, 187.3382) (-55.3103, 187.3972) (-55.6546, 187.8019) (-55.8272, 188.005) knots 0 0 0 0 0.076386 0.153256 0.153256 0.153256 0.153256
  line L104 (-55.8272, 188.005) -> (-55.8272, 187.4153)
  line L105 (-55.8272, 187.4153) -> (-56.5677, 187.4153)
  line L106 (-56.5677, 187.4153) -> (-56.5677, 193.9153)
  line L107 (-56.5677, 193.9153) -> (-55.7696, 193.9153)
  line L108 (-55.7696, 193.9153) -> (-55.7696, 191.5964)
  spline S51 degree 3 poles (-55.7696, 191.5964) (-55.5907, 191.7813) (-55.2364, 192.1477) (-54.7301, 192.203) (-54.4793, 192.2304) knots 0 0 0 0 0.074638 0.14787 0.14787 0.14787 0.14787
  spline S52 degree 3 poles (-54.4793, 192.2304) (-54.3368, 192.2233) (-54.0532, 192.2091) (-53.7885, 192.1064) (-53.6569, 192.0553) knots 0 0 0 0 0.042514 0.084577 0.084577 0.084577 0.084577
  spline S53 degree 3 poles (-53.6569, 192.0553) (-53.5338, 191.9917) (-53.2911, 191.8663) (-53.1085, 191.6633) (-53.0184, 191.5631) knots 0 0 0 0 0.041157 0.081209 0.081209 0.081209 0.081209
  spline S54 degree 3 poles (-53.0184, 191.5631) (-52.9386, 191.4493) (-52.7726, 191.2126) (-52.6761, 190.9399) (-52.626, 190.7983) knots 0 0 0 0 0.041496 0.086317 0.086317 0.086317 0.086317
  spline S55 degree 3 poles (-52.626, 190.7983) (-52.5846, 190.6447) (-52.5001, 190.3311) (-52.4895, 190.0063) (-52.4841, 189.8406) knots 0 0 0 0 0.04754 0.097104 0.097104 0.097104 0.097104
  spline S56 degree 3 poles (-52.4841, 189.8406) (-52.4995, 189.4713) (-52.528, 188.7899) (-52.9084, 188.2272) (-53.0827, 187.9695) knots 0 0 0 0 0.108337 0.199906 0.199906 0.199906 0.199906
  spline S57 degree 3 poles (-53.0827, 187.9695) (-53.2896, 187.7768) (-53.6964, 187.3982) (-54.2482, 187.3383) (-54.5192, 187.3089) knots 0 0 0 0 0.082403 0.16195 0.16195 0.16195 0.16195
  spline S58 degree 3 poles (-49.6021, 187.3089) (-49.9123, 187.3316) (-50.5128, 187.3757) (-50.9764, 187.758) (-51.2005, 187.9429) knots 0 0 0 0 0.090792 0.175782 0.175782 0.175782 0.175782
  spline S59 degree 3 poles (-51.2005, 187.9429) (-51.378, 188.192) (-51.7656, 188.7359) (-51.7945, 189.4063) (-51.8102, 189.7696) knots 0 0 0 0 0.089871 0.196272 0.196272 0.196272 0.196272
  spline S60 degree 3 poles (-51.8102, 189.7696) (-51.792, 190.166) (-51.7585, 190.8949) (-51.2947, 191.4527) (-51.083, 191.7072) knots 0 0 0 0 0.115281 0.212035 0.212035 0.212035 0.212035
  spline S61 degree 3 poles (-51.083, 191.7072) (-50.8662, 191.8598) (-50.422, 192.1723) (-49.8797, 192.2108) (-49.6021, 192.2304) knots 0 0 0 0 0.077985 0.159734 0.159734 0.159734 0.159734
  spline S62 degree 3 poles (-49.6021, 192.2304) (-49.296, 192.2068) (-48.6994, 192.1607) (-48.239, 191.7797) (-48.0148, 191.5942) knots 0 0 0 0 0.089656 0.174785 0.174785 0.174785 0.174785
  spline S63 degree 3 poles (-48.0148, 191.5942) (-47.8353, 191.3509) (-47.4509, 190.8303) (-47.4167, 190.1817) (-47.3985, 189.8362) knots 0 0 0 0 0.08875 0.189968 0.189968 0.189968 0.189968
  spline S64 degree 3 poles (-47.3985, 189.8362) (-47.4038, 189.5619) (-47.4134, 189.0687) (-47.5919, 188.61) (-47.6712, 188.4062) knots 0 0 0 0 0.08148 0.146573 0.146573 0.146573 0.146573
  spline S65 degree 3 poles (-47.6712, 188.4062) (-47.7727, 188.2421) (-47.9764, 187.9128) (-48.3017, 187.7025) (-48.4648, 187.5971) knots 0 0 0 0 0.057116 0.114612 0.114612 0.114612 0.114612
  spline S66 degree 3 poles (-48.4648, 187.5971) (-48.6434, 187.513) (-49.0037, 187.3434) (-49.4015, 187.3204) (-49.6021, 187.3089) knots 0 0 0 0 0.058612 0.118296 0.118296 0.118296 0.118296
  spline S67 degree 3 poles (-59.7024, 187.3089) (-60.0126, 187.3316) (-60.6131, 187.3757) (-61.0766, 187.758) (-61.3008, 187.9429) knots 0 0 0 0 0.090792 0.175782 0.175782 0.175782 0.175782
  spline S68 degree 3 poles (-61.3008, 187.9429) (-61.4783, 188.192) (-61.8659, 188.7359) (-61.8948, 189.4063) (-61.9104, 189.7696) knots 0 0 0 0 0.089871 0.196272 0.196272 0.196272 0.196272
  spline S69 degree 3 poles (-61.9104, 189.7696) (-61.8922, 190.166) (-61.8588, 190.8949) (-61.3949, 191.4527) (-61.1833, 191.7072) knots 0 0 0 0 0.115281 0.212035 0.212035 0.212035 0.212035
  spline S70 degree 3 poles (-61.1833, 191.7072) (-60.9664, 191.8598) (-60.5223, 192.1723) (-59.9799, 192.2108) (-59.7024, 192.2304) knots 0 0 0 0 0.077985 0.159734 0.159734 0.159734 0.159734
  spline S71 degree 3 poles (-59.7024, 192.2304) (-59.3963, 192.2068) (-58.7996, 192.1607) (-58.3393, 191.7797) (-58.1151, 191.5942) knots 0 0 0 0 0.089656 0.174785 0.174785 0.174785 0.174785
  spline S72 degree 3 poles (-58.1151, 191.5942) (-57.9355, 191.3509) (-57.5512, 190.8303) (-57.517, 190.1817) (-57.4988, 189.8362) knots 0 0 0 0 0.08875 0.189968 0.189968 0.189968 0.189968
  spline S73 degree 3 poles (-57.4988, 189.8362) (-57.5041, 189.5619) (-57.5137, 189.0687) (-57.6922, 188.61) (-57.7715, 188.4062) knots 0 0 0 0 0.08148 0.146573 0.146573 0.146573 0.146573
  spline S74 degree 3 poles (-57.7715, 188.4062) (-57.873, 188.2421) (-58.0767, 187.9128) (-58.4019, 187.7025) (-58.5651, 187.5971) knots 0 0 0 0 0.057116 0.114612 0.114612 0.114612 0.114612
  spline S75 degree 3 poles (-58.5651, 187.5971) (-58.7437, 187.513) (-59.104, 187.3434) (-59.5017, 187.3204) (-59.7024, 187.3089) knots 0 0 0 0 0.058612 0.118295 0.118295 0.118295 0.118295
  line L109 (-45.6693, 200.1315) -> (-45.6693, 197.5599)
  line L110 (-45.6693, 197.5599) -> (-46.4674, 197.5599)
  line L111 (-46.4674, 197.5599) -> (-46.4674, 202.2686)
  line L112 (-46.4674, 202.2686) -> (-45.7491, 202.2686)
  line L113 (-45.7491, 202.2686) -> (-45.7491, 201.5991)
  spline S76 degree 3 poles (-45.7491, 201.5991) (-45.5547, 201.8254) (-45.16, 202.2847) (-44.5566, 202.3446) (-44.2505, 202.375) knots 0 0 0 0 0.086062 0.174671 0.174671 0.174671 0.174671
  spline S77 degree 3 poles (-44.2505, 202.375) (-44.1129, 202.3693) (-43.8442, 202.3581) (-43.5913, 202.2667) (-43.4679, 202.2221) knots 0 0 0 0 0.041025 0.080156 0.080156 0.080156 0.080156
  spline S78 degree 3 poles (-43.4679, 202.2221) (-43.3586, 202.1701) (-43.153, 202.0722) (-43.0036, 201.901) (-42.9336, 201.8208) knots 0 0 0 0 0.035864 0.067451 0.067451 0.067451 0.067451
  spline S79 degree 3 poles (-42.9336, 201.8208) (-42.8786, 201.7323) (-42.7645, 201.5491) (-42.7123, 201.3395) (-42.6853, 201.2311) knots 0 0 0 0 0.031061 0.064335 0.064335 0.064335 0.064335
  spline S80 degree 3 poles (-42.6853, 201.2311) (-42.6725, 201.1296) (-42.6401, 200.8721) (-42.6407, 200.6125) (-42.641, 200.4552) knots 0 0 0 0 0.030663 0.077786 0.077786 0.077786 0.077786
  line L114 (-42.641, 200.4552) -> (-42.641, 197.5599)
  line L115 (-42.641, 197.5599) -> (-43.4391, 197.5599)
  line L116 (-43.4391, 197.5599) -> (-43.4391, 200.4241)
  spline S81 degree 3 poles (-43.4391, 200.4241) (-43.4399, 200.5672) (-43.4412, 200.8145) (-43.5052, 201.053) (-43.5322, 201.1535) knots 0 0 0 0 0.042684 0.073794 0.073794 0.073794 0.073794
  spline S82 degree 3 poles (-43.5322, 201.1535) (-43.57, 201.2304) (-43.6469, 201.3872) (-43.7898, 201.4879) (-43.8625, 201.5393) knots 0 0 0 0 0.025274 0.051516 0.051516 0.051516 0.051516
  spline S83 degree 3 poles (-43.8625, 201.5393) (-43.9468, 201.5813) (-44.122, 201.6685) (-44.3176, 201.6783) (-44.419, 201.6834) knots 0 0 0 0 0.027946 0.058036 0.058036 0.058036 0.058036
  spline S84 degree 3 poles (-44.419, 201.6834) (-44.5825, 201.6704) (-44.9063, 201.6448) (-45.169, 201.4541) (-45.2991, 201.3597) knots 0 0 0 0 0.048182 0.095412 0.095412 0.095412 0.095412
  spline S85 degree 3 poles (-45.2991, 201.3597) (-45.4063, 201.2084) (-45.6641, 200.8447) (-45.6674, 200.3945) (-45.6693, 200.1315) knots 0 0 0 0 0.054493 0.130984 0.130984 0.130984 0.130984
  line L117 (-47.6823, 202.2686) -> (-47.6823, 197.5599)
  line L118 (-47.6823, 197.5599) -> (-48.4804, 197.5599)
  line L119 (-48.4804, 197.5599) -> (-48.4804, 202.2686)
  line L120 (-48.4804, 202.2686) -> (-47.6823, 202.2686)
  line L121 (-52.7368, 200.1359) -> (-52.7368, 197.5599)
  line L122 (-52.7368, 197.5599) -> (-53.5349, 197.5599)
  line L123 (-53.5349, 197.5599) -> (-53.5349, 204.0599)
  line L124 (-53.5349, 204.0599) -> (-52.7368, 204.0599)
  line L125 (-52.7368, 204.0599) -> (-52.7368, 201.7277)
  spline S86 degree 3 poles (-52.7368, 201.7277) (-52.5386, 201.9165) (-52.1426, 202.2936) (-51.5986, 202.3479) (-51.3269, 202.375) knots 0 0 0 0 0.079682 0.15916 0.15916 0.15916 0.15916
  spline S87 degree 3 poles (-51.3269, 202.375) (-51.1615, 202.3682) (-50.8456, 202.355) (-50.556, 202.229) (-50.4179, 202.1689) knots 0 0 0 0 0.049154 0.09392 0.09392 0.09392 0.09392
  spline S88 degree 3 poles (-50.4179, 202.1689) (-50.2992, 202.0951) (-50.0674, 201.9511) (-49.932, 201.7145) (-49.8659, 201.5991) knots 0 0 0 0 0.041202 0.080448 0.080448 0.080448 0.080448
  spline S89 degree 3 poles (-49.8659, 201.5991) (-49.8177, 201.4517) (-49.7057, 201.1097) (-49.7018, 200.7491) (-49.6997, 200.5439) knots 0 0 0 0 0.046272 0.107379 0.107379 0.107379 0.107379
  line L126 (-49.6997, 200.5439) -> (-49.6997, 197.5599)
  line L127 (-49.6997, 197.5599) -> (-50.4977, 197.5599)
  line L128 (-50.4977, 197.5599) -> (-50.4977, 200.5439)
  spline S90 degree 3 poles (-50.4977, 200.5439) (-50.5019, 200.7219) (-50.5093, 201.038) (-50.6818, 201.3005) (-50.7571, 201.4151) knots 0 0 0 0 0.052115 0.092521 0.092521 0.092521 0.092521
  spline S91 degree 3 poles (-50.7571, 201.4151) (-50.8571, 201.4946) (-51.0711, 201.6645) (-51.345, 201.6797) (-51.4909, 201.6878) knots 0 0 0 0 0.037401 0.080016 0.080016 0.080016 0.080016
  spline S92 degree 3 poles (-51.4909, 201.6878) (-51.6077, 201.6799) (-51.8427, 201.6642) (-52.0526, 201.5575) (-52.1582, 201.5038) knots 0 0 0 0 0.034724 0.069859 0.069859 0.069859 0.069859
  spline S93 degree 3 poles (-52.1582, 201.5038) (-52.2546, 201.4379) (-52.4442, 201.3081) (-52.5512, 201.1049) (-52.6038, 201.005) knots 0 0 0 0 0.034441 0.067793 0.067793 0.067793 0.067793
  spline S94 degree 3 poles (-52.6038, 201.005) (-52.6425, 200.881) (-52.7305, 200.5985) (-52.7346, 200.3022) (-52.7368, 200.1359) knots 0 0 0 0 0.038771 0.08832 0.08832 0.08832 0.08832
  spline S95 degree 3 poles (-59.126, 198.1097) (-58.9869, 198.1179) (-58.718, 198.1338) (-58.4878, 198.273) (-58.3767, 198.3402) knots 0 0 0 0 0.041087 0.079456 0.079456 0.079456 0.079456
  spline S96 degree 3 poles (-58.3767, 198.3402) (-58.2764, 198.4349) (-58.0569, 198.6421) (-57.9452, 198.9234) (-57.8845, 199.0763) knots 0 0 0 0 0.040863 0.089495 0.089495 0.089495 0.089495
  line L129 (-57.8845, 199.0763) -> (-57.0598, 198.9743)
  spline S97 degree 3 poles (-57.0598, 198.9743) (-57.1356, 198.7493) (-57.2822, 198.3139) (-57.6195, 198.0028) (-57.7825, 197.8525) knots 0 0 0 0 0.069951 0.135368 0.135368 0.135368 0.135368
  spline S98 degree 3 poles (-57.7825, 197.8525) (-57.9777, 197.7362) (-58.3921, 197.4894) (-58.875, 197.4659) (-59.1304, 197.4535) knots 0 0 0 0 0.06712 0.142493 0.142493 0.142493 0.142493
  spline S99 degree 3 poles (-59.1304, 197.4535) (-59.4518, 197.4748) (-60.0664, 197.5155) (-60.5419, 197.9043) (-60.7687, 198.0897) knots 0 0 0 0 0.093968 0.179695 0.179695 0.179695 0.179695
  spline S100 degree 3 poles (-60.7687, 198.0897) (-60.945, 198.3356) (-61.3258, 198.8668) (-61.3571, 199.5223) (-61.3739, 199.8744) knots 0 0 0 0 0.088891 0.192041 0.192041 0.192041 0.192041
  spline S101 degree 3 poles (-61.3739, 199.8744) (-61.3573, 200.2381) (-61.3265, 200.9133) (-60.9403, 201.4645) (-60.7621, 201.7188) knots 0 0 0 0 0.106628 0.197922 0.197922 0.197922 0.197922
  spline S102 degree 3 poles (-60.7621, 201.7188) (-60.5393, 201.9102) (-60.0829, 202.3022) (-59.4822, 202.3504) (-59.1748, 202.375) knots 0 0 0 0 0.085796 0.175759 0.175759 0.175759 0.175759
  spline S103 degree 3 poles (-59.1748, 202.375) (-58.8765, 202.3505) (-58.292, 202.3025) (-57.8488, 201.9196) (-57.6318, 201.7321) knots 0 0 0 0 0.087287 0.171058 0.171058 0.171058 0.171058
  spline S104 degree 3 poles (-57.6318, 201.7321) (-57.4575, 201.4828) (-57.0794, 200.9419) (-57.0494, 200.28) (-57.0332, 199.9231) knots 0 0 0 0 0.089451 0.194057 0.194057 0.194057 0.194057
  spline S105 degree 3 poles (-57.0332, 199.9231) (-57.0335, 199.8936) (-57.0342, 199.8226) (-57.0364, 199.7517) (-57.0377, 199.7103) knots 0 0 0 0 0.008868 0.021288 0.021288 0.021288 0.021288
  line L130 (-57.0377, 199.7103) -> (-60.5493, 199.7103)
  spline S106 degree 3 poles (-60.5493, 199.7103) (-60.5262, 199.4739) (-60.4836, 199.0377) (-60.2276, 198.684) (-60.1103, 198.522) knots 0 0 0 0 0.069761 0.128713 0.128713 0.128713 0.128713
  spline S107 degree 3 poles (-60.1103, 198.522) (-59.9697, 198.4018) (-59.686, 198.159) (-59.3138, 198.1262) (-59.126, 198.1097) knots 0 0 0 0 0.054058 0.109125 0.109125 0.109125 0.109125
  line L131 (-100, 145) -> (-80, 155)
  line L132 (-80, 155) -> (-80, 160)
  line L133 (-80, 160) -> (-100, 150)
  line L134 (-100, 150) -> (-100, 145)
  line L135 (-105, 145) -> (-105, 150)
  line L136 (-105, 150) -> (-125, 160)
  line L137 (-125, 160) -> (-125, 155)
  line L138 (-125, 155) -> (-105, 145)
  line L139 (-100, 155) -> (-80, 165)
  line L140 (-80, 165) -> (-80, 170)
  line L141 (-80, 170) -> (-100, 160)
  line L142 (-100, 160) -> (-100, 155)
  line L143 (-105, 155) -> (-105, 160)
  line L144 (-105, 160) -> (-125, 170)
  line L145 (-125, 170) -> (-125, 165)
  line L146 (-125, 165) -> (-105, 155)
  line L147 (-100, 165) -> (-80, 175)
  line L148 (-80, 175) -> (-80, 180)
  line L149 (-80, 180) -> (-100, 170)
  line L150 (-100, 170) -> (-100, 165)
  line L151 (-105, 165) -> (-105, 170)
  line L152 (-105, 170) -> (-125, 180)
  line L153 (-125, 180) -> (-125, 175)
  line L154 (-125, 175) -> (-105, 165)
  line L155 (-100, 175) -> (-80, 185)
  line L156 (-80, 185) -> (-80, 190)
  line L157 (-80, 190) -> (-100, 180)
  line L158 (-100, 180) -> (-100, 175)
  line L159 (-105, 175) -> (-105, 180)
  line L160 (-105, 180) -> (-125, 190)
  line L161 (-125, 190) -> (-125, 185)
  line L162 (-125, 185) -> (-105, 175)
  line L163 (-100, 185) -> (-80, 195)
  line L164 (-80, 195) -> (-80, 200)
  line L165 (-80, 200) -> (-100, 190)
  line L166 (-100, 190) -> (-100, 185)
  line L167 (-105, 185) -> (-105, 190)
  line L168 (-105, 190) -> (-125, 200)
  line L169 (-125, 200) -> (-125, 195)
  line L170 (-125, 195) -> (-105, 185)
  line L171 (-100, 195) -> (-80, 205)
  line L172 (-80, 205) -> (-80, 210)
  line L173 (-80, 210) -> (-100, 200)
  line L174 (-100, 200) -> (-100, 195)
  line L175 (-105, 195) -> (-105, 200)
  line L176 (-105, 200) -> (-125, 210)
  line L177 (-125, 210) -> (-125, 205)